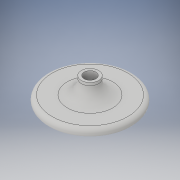
# Autodesk Inventor part: Front Wheel
Saved by Autodesk Inventor 2018 (Build 220112000, 112)
## iProperties
Created: 2018-02-14
Part Number: Front Wheel
Material: Generic
Document SubType Name: Modeling
Designer: Karin
Density: 1 g/cm^3
Appearance: Default
Author: Karin
Autodesk Inventor part; units mm, degrees
ref_plane "YZ Plane" through (0, 0, 0) normal (1, 0, 0) x (0, 1, 0)
ref_plane "XZ Plane" through (0, 0, 0) normal (0, 1, 0) x (-1, 0, 0)
ref_plane "XY Plane" through (0, 0, 0) normal (0, 0, 1) x (1, 0, 0)
sketch "Sketch1" plane through (0, 0, 0) normal (0, 0, 1) x (1, 0, 0)
  line L0 (2.667, 0) -> (19.05, 0)
  line L1 (19.05, 0) -> (19.05, 3.81)
  line L2 (19.05, 3.81) -> (3.937, 3.81)
  line L3 (3.937, 3.81) -> (3.937, 11.43)
  line L4 (3.937, 11.43) -> (2.667, 11.43)
  line L5 (2.667, 11.43) -> (2.667, 0)
  line L6 (0, 25.5419) -> (0, -2.7317)
  point P0 (0, 0)
  dimension "d11" = 19.05
  dimension "d12" = 3.81
  dimension "d13" = 1.27
  dimension "d15" = 2.667
  dimension "d16" = 7.62
  constraints: 14 end point, 5 perpendicular, 1 horizontal, 1 vertical
  measures "d11" distance of point (0, 0) L0.end
  measures "d12" distance of L0.end L1.end
  measures "d13" distance of L3.end L4.end
  measures "d15" distance from line of point (0, 0) L5
  measures "d16" distance of L2.end L3.end
revolve "Revolution1" add sketch "Sketch1" angle 360 about axis through (0, 25.5419, 0) along (0, -1, 0)
fillet "Fillet1" radius 6.35 1 edges at (-3.937, 3.81, 0)
fillet "Fillet2" radius 1.905 2 edges at (-19.05, 3.81, 0) (-19.05, 0, 0)
body "Solid1"
